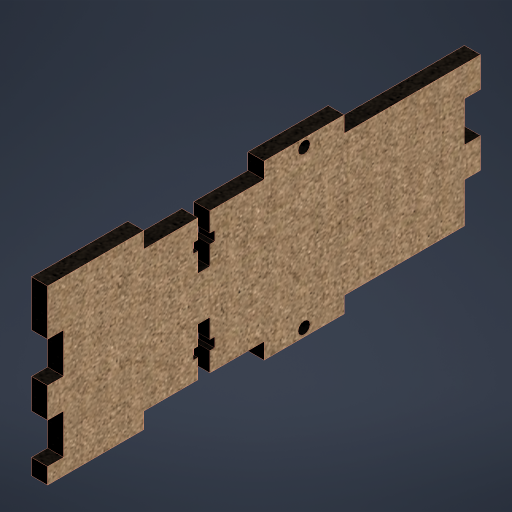
# Autodesk Inventor part: FloorButtonHolder_Side_V1
Saved by Autodesk Inventor 2024.1 (Build 281209000, 209)
## iProperties
Created: 2023-05-20
Part Number: FloorButtonHolder_Side_V1
Material: MDF Medium Density Fiberboard
Document SubType Name: Modeling
Designer: jaege
Density: 0.8 g/cm^3
Appearance: Red Oak - Natural Low Gloss
Author: jaege
Autodesk Inventor part; units mm, degrees
ref_plane "YZ Plane" through (0, 0, 0) normal (1, 0, 0) x (0, 1, 0)
ref_plane "XZ Plane" through (0, 0, 0) normal (0, 1, 0) x (-1, 0, 0)
ref_plane "XY Plane" through (0, 0, 0) normal (0, 0, 1) x (1, 0, 0)
sketch "Sketch1" plane through (0, 0, 0) normal (1, 0, 0) x (0, 1, 0)
  line L0 (-17.5, 50) -> (17.5, 50)
  line L1 (17.5, 50) -> (17.5, -50)
  line L2 (17.5, -50) -> (-17.5, -50)
  line L3 (-17.5, -50) -> (-17.5, 50)
  line L4 (-17.5, 50) -> (17.5, -50) construction
  line L5 (17.5, 50) -> (-17.5, -50) construction
  line L6 (17.5, 50) -> (10, 50)
  line L7 (10, 50) -> (10, 54)
  line L8 (10, 54) -> (17.5, 54)
  line L9 (17.5, 54) -> (17.5, 50)
  line L10 (0, 50) -> (-7.5, 50)
  line L11 (-7.5, 50) -> (-7.5, 54)
  line L12 (-7.5, 54) -> (0, 54)
  line L13 (0, 54) -> (0, 50)
  line L14 (17.5, 0) -> (-17.5, 0) construction
  line L15 (0, 50) -> (0, -50) construction
  line L16 (17.5, -50) -> (10, -50)
  line L17 (10, -50) -> (10, -54)
  line L18 (10, -54) -> (17.5, -54)
  line L19 (17.5, -54) -> (17.5, -50)
  line L20 (0, -50) -> (-7.5, -50)
  line L21 (-7.5, -50) -> (-7.5, -54)
  line L22 (-7.5, -54) -> (0, -54)
  line L23 (0, -54) -> (0, -50)
  line L24 (17.5, 50) -> (21.5, 50)
  line L25 (21.5, 50) -> (21.5, 30)
  line L26 (21.5, 30) -> (17.5, 30)
  line L27 (17.5, 30) -> (17.5, 50)
  line L28 (17.5, 0) -> (21.5, 0)
  line L29 (21.5, 0) -> (21.5, -20)
  line L30 (21.5, -20) -> (17.5, -20)
  line L31 (17.5, -20) -> (17.5, 0)
  line L32 (-17.5, 0) -> (-21.5, 0)
  line L33 (-21.5, 0) -> (-21.5, -20)
  line L34 (-21.5, -20) -> (-17.5, -20)
  line L35 (-17.5, -20) -> (-17.5, 0)
  line L36 (17.5, 50) -> (21.5, 50)
  line L37 (21.5, 50) -> (21.5, 54)
  line L38 (21.5, 54) -> (17.5, 54)
  line L39 (17.5, 54) -> (17.5, 50)
  line L40 (-17.5, 30) -> (-21.5, 30)
  line L41 (-21.5, 30) -> (-21.5, 54)
  line L42 (-21.5, 54) -> (-17.5, 54)
  line L43 (-17.5, 54) -> (-17.5, 30)
  point P0 (0, 0)
  point P1 (0, 52)
  point P2 (0, -52)
  point P3 (-17.5, -20)
  point P4 (-7.5, -50)
  point P5 (10, -50)
  point P6 (17.5, -20)
  point P7 (17.5, 30)
  point P8 (10, 50)
  point P9 (-7.5, 50)
  point P10 (-19.5, 0)
  point P11 (-19.5, 30)
  dimension "d0" = 35
  dimension "d2" = 7.5
  dimension "d3" = 4
  dimension "d4" = 7.5
  dimension "d5" = 4
  dimension "d6" = 10
  dimension "d7" = 4
  dimension "d8" = 20
  dimension "d9" = 4
  dimension "d10" = 20
  dimension "d13" = 4
  dimension "d14" = 20
  dimension "d17" = 4
  dimension "d18" = 24
  dimension "d19" = 30
  constraints: 88 end point, 16 parallel, 9 midpoint, 8 horizontal, 8 perpendicular, 7 symmetric about line, 3 collinear, 1 point on line
  measures "d0" distance of L1.end L2.end
  measures "d2" distance of L7.end L8.end
  measures "d3" distance of L6.end L7.end
  measures "d4" distance of L11.end L12.end
  measures "d5" distance of L10.end L11.end
  measures "d6" distance from line of point (0, 52) L7
  measures "d7" distance of L25.end L26.end
  measures "d8" distance of L24.end L25.end
  measures "d9" distance of L29.end L30.end
  measures "d10" distance of L28.end L29.end
  measures "d13" distance of L34.end L33.end
  measures "d14" distance of L33.end L32.end
  measures "d17" distance of L41.end L42.end
  measures "d18" distance of L40.end L41.end
  measures "d19" distance of point (-19.5, 0) point (-19.5, 30)
extrude "Extrusion1" add sketch "Sketch1" along normal blind 4
sketch "Sketch2" plane through (0, 0, 0) normal (-1, 0, 0) x (0, 0, 1)
  line L0 (-8.5, 17.5) -> (-11.5, 17.5) construction
  line L1 (-8.5, 21.5) -> (-8.5, 17.5) construction
  line L2 (-11.5, 21.5) -> (-8.5, 21.5) construction
  line L3 (-11.5, 21.5) -> (-11.5, 17.5) construction
  line L4 (13.5, 21.5) -> (16.5, 21.5) projected
  line L5 (-11.5, 21.5) -> (-8.5, 17.5) construction
  circle A0 centre (-10, 19.5) radius 1.5
  line L6 (13.5, 17.5) -> (16.5, 17.5)
  line L7 (16.5, 17.5) -> (16.5, 5.5)
  line L8 (16.5, 5.5) -> (13.5, 5.5)
  line L9 (13.5, 5.5) -> (13.5, 17.5)
  line L10 (0, 17.5) -> (30, 17.5) projected
  line L11 (12.3, 10.3) -> (17.7, 10.3)
  line L12 (17.7, 10.3) -> (17.7, 12.7)
  line L13 (17.7, 12.7) -> (12.3, 12.7)
  line L14 (12.3, 12.7) -> (12.3, 10.3)
  line L15 (13.5, -5.5) -> (16.5, -5.5)
  line L16 (16.5, -5.5) -> (16.5, -17.5)
  line L17 (16.5, -17.5) -> (13.5, -17.5)
  line L18 (13.5, -17.5) -> (13.5, -5.5)
  line L19 (12.3, -12.7) -> (17.7, -12.7)
  line L20 (17.7, -12.7) -> (17.7, -10.3)
  line L21 (17.7, -10.3) -> (12.3, -10.3)
  line L22 (12.3, -10.3) -> (12.3, -12.7)
  line L23 (30, -17.5) -> (0, -17.5) projected
  line L24 (16.5, -21.5) -> (13.5, -21.5) projected
  line L25 (30, 21.5) -> (54, 21.5) construction
  line L26 (54, 21.5) -> (54, 10) construction
  line L27 (54, 10) -> (50, 10) construction
  line L28 (50, 10) -> (50, 0) construction
  line L29 (50, 0) -> (54, 0) construction
  line L30 (54, 0) -> (54, -7.5) construction
  line L31 (54, -7.5) -> (50, -7.5) construction
  line L32 (50, -7.5) -> (50, -17.5) construction
  line L33 (50, -17.5) -> (54, -17.5) construction
  line L34 (54, -17.5) -> (54, -21.5) construction
  line L35 (54, -21.5) -> (30, -21.5) construction
  line L36 (30, -21.5) -> (30, -17.5) construction
  line L37 (30, -17.5) -> (0, -17.5) construction
  line L38 (0, -17.5) -> (0, -21.5) construction
  line L39 (0, -21.5) -> (-20, -21.5) construction
  line L40 (-20, -21.5) -> (-20, -17.5) construction
  line L41 (-20, -17.5) -> (-50, -17.5) construction
  line L42 (-50, -17.5) -> (-50, -7.5) construction
  line L43 (-50, -7.5) -> (-54, -7.5) construction
  line L44 (-54, -7.5) -> (-54, 0) construction
  line L45 (-54, 0) -> (-50, 0) construction
  line L46 (-50, 0) -> (-50, 10) construction
  line L47 (-50, 10) -> (-54, 10) construction
  line L48 (-54, 10) -> (-54, 17.5) construction
  line L49 (-54, 17.5) -> (-20, 17.5) construction
  line L50 (-20, 17.5) -> (-20, 21.5) construction
  line L51 (-20, 21.5) -> (0, 21.5) construction
  line L52 (0, 21.5) -> (0, 17.5) construction
  line L53 (0, 17.5) -> (30, 17.5) construction
  line L54 (30, 17.5) -> (30, 21.5) construction
  line L55 (-11.5, -17.5) -> (-8.5, -17.5) construction
  line L56 (-11.5, -21.5) -> (-11.5, -17.5) construction
  line L57 (-8.5, -21.5) -> (-11.5, -21.5) construction
  line L58 (-8.5, -21.5) -> (-8.5, -17.5) construction
  line L59 (-11.5, -17.5) -> (-8.5, -21.5) construction
  circle A1 centre (-10, -19.5) radius 1.5
  point P0 (0, 0)
  point P1 (15, 17.5)
  point P2 (15, 21.5)
  point P3 (15, 12.7)
  point P4 (17.7, 11.5)
  point P5 (16.5, 11.5)
  point P6 (15, -5.5)
  point P7 (15, -10.3)
  point P8 (17.7, -11.5)
  point P9 (16.5, -11.5)
  point P10 (15, -21.5)
  point P11 (16.5, 12.7)
  point P12 (13.5, 12.7)
  point P13 (13.5, 10.3)
  point P14 (16.5, 10.3)
  point P15 (13.5, -10.3)
  point P16 (13.5, -12.7)
  point P17 (16.5, -12.7)
  point P18 (16.5, -10.3)
  dimension "d20" = 3
  dimension "d21" = 3
  dimension "d22" = 12
  dimension "d23" = 5.4
  dimension "d24" = 2.4
  dimension "d25" = 3
  dimension "d26" = 12
  dimension "d27" = 5.4
  dimension "d28" = 2.4
  dimension "d31" = 3
  constraints: 36 end point, 13 midpoint, 8 parallel, 4 horizontal, 4 horizontal alignment, 4 perpendicular, 4 vertical alignment, 2 centre point, 1 other
  measures "d20" diameter of A0
  measures "d21" distance of L7.end L8.end
  measures "d22" distance of L8.end L6.start
  measures "d23" distance of L12.end L13.end
  measures "d24" distance of L11.end L12.end
  measures "d25" distance of L17.start L18.start
  measures "d26" distance of L18.start L15.start
  measures "d27" distance of L20.end L22.start
  measures "d28" distance of L19.end L20.end
  measures "d31" diameter of A1
extrude "Extrusion2" cut sketch "Sketch2" against normal up to next
body "Solid1"
